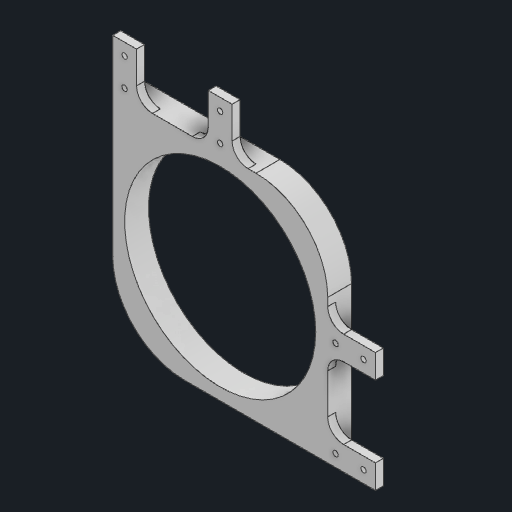
# Autodesk Inventor part: Midplate
Saved by Autodesk Inventor 2023 (Build 270158000, 158)
## iProperties
Created: 2022-11-11
Part Number: Midplate
Material: Generic
Document SubType Name: Modeling
Designer: izack
Density: 1 g/cm^3
Appearance: Default
Author: izack
Autodesk Inventor part; units mm, degrees
ref_plane "YZ Plane" through (0, 0, 0) normal (1, 0, 0) x (0, 1, 0)
ref_plane "XZ Plane" through (0, 0, 0) normal (0, 1, 0) x (-1, 0, 0)
ref_plane "XY Plane" through (0, 0, 0) normal (0, 0, 1) x (1, 0, 0)
sketch "Sketch1" plane through (0, 0, 0) normal (0, 0, 1) x (1, 0, 0)
  circle A0 centre (-0.5847, 59.562) radius 8.65 projected
  circle A1 centre (-0.5847, 59.562) radius 59.9665
  line L0 (-23.0847, -7.938) -> (21.9153, -7.938)
  line L1 (66.9153, 82.062) -> (66.9153, 82.062)
  line L2 (21.9153, 127.062) -> (21.9153, 127.062)
  line L3 (-68.0847, 82.062) -> (-68.0847, 37.062)
  line L4 (-68.0847, -7.938) -> (66.9153, 127.062) construction
  line L5 (66.9153, -7.938) -> (-68.0847, 127.062) construction
  arc A2 (-68.0847, 37.062) -> (-23.0847, -7.938) centre (-23.0847, 37.062) ccw
  arc A3 (66.9153, 82.062) -> (21.9153, 127.062) centre (21.9153, 82.062) ccw
  circle A4 centre (-0.5847, 59.562) radius 67.5
  line L6 (-18.0847, 127.062) -> (-23.0847, 127.062)
  line L7 (66.9153, 42.062) -> (66.9153, 37.062)
  arc A5 (-23.0847, 127.062) -> (-68.0847, 82.062) centre (-23.0847, 82.062) ccw
  arc A6 (21.9153, -7.938) -> (66.9153, 37.062) centre (21.9153, 37.062) ccw
  line L8 (21.9153, -7.938) -> (66.9153, -7.938)
  line L9 (66.9153, 37.062) -> (66.9153, 17.062)
  line L10 (-68.0847, 82.062) -> (-68.0847, 127.062)
  line L11 (-23.0847, 127.062) -> (-43.0847, 127.062)
  line L12 (-68.0847, 127.062) -> (-68.0847, 157.062)
  line L13 (-68.0847, 157.062) -> (-53.0847, 157.062)
  line L14 (-53.0847, 157.062) -> (-53.0847, 137.062)
  line L15 (66.9153, -7.938) -> (96.9153, -7.938)
  line L16 (96.9153, -7.938) -> (96.9153, 7.062)
  line L17 (96.9153, 7.062) -> (76.9153, 7.062)
  arc A7 (-53.0847, 137.062) -> (-43.0847, 127.062) centre (-43.0847, 137.062) ccw
  arc A8 (66.9153, 17.062) -> (76.9153, 7.062) centre (76.9153, 17.062) ccw
  line L18 (-0.5847, 59.562) -> (66.9153, 39.562) construction
  line L19 (76.9153, 67.062) -> (96.9153, 67.062)
  line L20 (96.9153, 67.062) -> (96.9153, 52.062)
  line L21 (96.9153, 52.062) -> (76.9153, 52.062)
  arc A9 (76.9153, 52.062) -> (66.9153, 42.062) centre (76.9153, 42.062) ccw
  line L22 (66.9153, 82.062) -> (66.9153, 77.062)
  arc A10 (66.9153, 77.062) -> (76.9153, 67.062) centre (76.9153, 77.062) ccw
  line L23 (-8.0847, 137.062) -> (-8.0847, 157.062)
  line L24 (-8.0847, 157.062) -> (6.9153, 157.062)
  line L25 (6.9153, 157.062) -> (6.9153, 137.062)
  arc A11 (-18.0847, 127.062) -> (-8.0847, 137.062) centre (-18.0847, 137.062) ccw
  line L26 (21.9153, 127.062) -> (16.9153, 127.062)
  arc A12 (6.9153, 137.062) -> (16.9153, 127.062) centre (16.9153, 137.062) ccw
  line L27 (-60.5847, 157.062) -> (-60.5847, 106.9366) construction
  line L28 (-0.5847, 157.062) -> (-0.5847, 127.062) construction
  line L29 (96.9153, 59.562) -> (66.9153, 59.612) construction
  line L30 (96.9153, -0.438) -> (46.9153, -0.3546) construction
  circle A13 centre (89.4153, -0.4255) radius 1.7
  circle A14 centre (71.9153, -0.3963) radius 1.7
  circle A15 centre (89.4153, 59.5745) radius 1.7
  circle A16 centre (71.9153, 59.6037) radius 1.7
  circle A17 centre (-0.5847, 132.062) radius 1.7
  circle A18 centre (-0.5847, 149.562) radius 1.7
  circle A19 centre (-60.5847, 149.562) radius 1.7
  circle A20 centre (-60.5847, 132.062) radius 1.7
  point P0 (0, 0)
  point P1 (21.9167, 127.0604)
  point P2 (66.9153, 67.062)
  point P3 (-8.0847, 127.062)
  point P4 (6.9153, 127.062)
  dimension "d0" = 119.933
  dimension "d1" = 135
  dimension "d2" = 135
  dimension "d10" = 45
  dimension "d33" = 45
  dimension "d34" = 30
  dimension "d35" = 15
  dimension "d36" = 30
  dimension "d37" = 10
  dimension "d38" = 30
  dimension "d39" = 15
  dimension "d41" = 45
  dimension "d42" = 15
  dimension "d43" = 10
  dimension "d44" = 10
  dimension "d45" = 30
  dimension "d46" = 15
  dimension "d47" = 45
  dimension "d48" = 10
  dimension "d49" = 10
  dimension "d50" = 3.4
  dimension "d51" = 3.4
  dimension "d52" = 3.4
  dimension "d53" = 3.4
  dimension "d54" = 3.4
  dimension "d55" = 3.4
  dimension "d56" = 3.4
  dimension "d57" = 3.4
  dimension "d58" = 7.5
  dimension "d59" = 25
  dimension "d60" = 7.5
  dimension "d61" = 25
  dimension "d62" = 25
  dimension "d63" = 7.5
  dimension "d64" = 7.5
  dimension "d65" = 25
  constraints: 62 end point, 30 point on line, 26 point on circle, 25 tangent, 20 centre point, 13 perpendicular, 8 midpoint, 5 horizontal, 4 parallel, 3 equal radius, 2 coincident, 2 vertical
  measures "d0" diameter of A1
  measures "d1" distance of L5.end L4.end
  measures "d2" distance of L4.end L5.start
  measures "d10" radius of A2
  measures "d33" radius of A5
  measures "d34" distance of L12.start L12.end
  measures "d35" distance of L12.end L13.end
  measures "d36" distance of L5.start L15.end
  measures "d37" radius of A7
  measures "d38" distance of point (66.915, 67.062) L19.end
  measures "d39" distance of L19.end L20.end
  measures "d41" distance between parallel lines of L21 L17
  measures "d42" distance between parallel lines of L15 L17
  measures "d43" radius of A9
  measures "d44" radius of A10
  measures "d45" distance of point (-8.085, 127.062) L23.end
  measures "d46" distance of L23.end L24.end
  measures "d47" distance between parallel lines of L14 L23
  measures "d48" radius of A11
  measures "d49" radius of A12
  measures "d50" diameter of A13
  measures "d51" diameter of A14
  measures "d52" diameter of A15
  measures "d53" diameter of A16
  measures "d54" diameter of A17
  measures "d55" diameter of A18
  measures "d56" diameter of A19
  measures "d57" diameter of A20
  measures "d58" distance from line of A13.centre L16
  measures "d59" distance from line of A14.centre L16
  measures "d60" distance from line of A15.centre L20
  measures "d61" distance from line of A16.centre L20
  measures "d62" distance from line of L24 A17.centre
  measures "d63" distance from line of L24 A18.centre
  measures "d64" distance from line of L13 A19.centre
  measures "d65" distance from line of L13 A20.centre
extrude "Extrusion1" add sketch "Sketch1" against normal blind 5 contours A2 L3 A4 L0 | A4 L3 A5 L6 A11 L23 L24 L25 A12 L26 A3 L22 A10 L19 L20 L21 A9 L7 A6 L0 | A4 | A6 L9 A8 L17 L16 L15 L8 | L10 L12 L13 L14 A7 L11 A5
sketch "Sketch2" plane through (0, 0, 0) normal (0, 0, 1) x (1, 0, 0)
  circle A0 centre (-0.5847, 59.562) radius 59.9665 projected
  circle A1 centre (-0.5847, 59.562) radius 67.5
  line L0 (96.9153, -7.938) -> (-23.0847, -7.938) projected
  line L1 (-68.0847, 127.062) -> (-68.0847, 37.062) projected
  arc A2 (-68.0847, 37.062) -> (-23.0847, -7.938) centre (-23.0847, 37.062) ccw projected
  line L2 (-23.0847, -7.938) -> (-68.0847, -7.938) projected
  circle A3 centre (-0.5847, 59.562) radius 56.9665
  line L3 (-18.0847, 127.062) -> (-43.0847, 127.062) projected
  arc A4 (-68.0847, 37.062) -> (-23.0847, -7.938) centre (-23.0847, 37.062) ccw projected
  arc A5 (66.9153, 82.062) -> (21.9153, 127.062) centre (21.9153, 82.062) ccw projected
  circle A6 centre (-0.5847, 59.562) radius 59.9665 projected
  arc A7 (76.9153, 52.062) -> (66.9153, 42.062) centre (76.9153, 42.062) ccw projected
  line L4 (76.9153, 52.062) -> (96.9153, 52.062) projected
  line L5 (96.9153, 52.062) -> (96.9153, 67.062) projected
  line L6 (96.9153, 67.062) -> (76.9153, 67.062) projected
  arc A8 (66.9153, 77.062) -> (76.9153, 67.062) centre (76.9153, 77.062) ccw projected
  line L7 (66.9153, 77.062) -> (66.9153, 82.062) projected
  line L8 (21.9153, 127.062) -> (16.9153, 127.062) projected
  arc A9 (6.9153, 137.062) -> (16.9153, 127.062) centre (16.9153, 137.062) ccw projected
  line L9 (6.9153, 137.062) -> (6.9153, 157.062) projected
  line L10 (6.9153, 157.062) -> (-8.0847, 157.062) projected
  line L11 (-8.0847, 157.062) -> (-8.0847, 137.062) projected
  arc A10 (-18.0847, 127.062) -> (-8.0847, 137.062) centre (-18.0847, 137.062) ccw projected
  line L12 (-68.0847, 157.062) -> (-68.0847, 37.062) projected
  line L13 (-23.0847, -7.938) -> (96.9153, -7.938) projected
  line L14 (96.9153, -7.938) -> (96.9153, 7.062) projected
  line L15 (96.9153, 7.062) -> (76.9153, 7.062) projected
  arc A11 (66.9153, 17.062) -> (76.9153, 7.062) centre (76.9153, 17.062) ccw projected
  line L16 (66.9153, 17.062) -> (66.9153, 42.062) projected
  arc A12 (-53.0847, 137.062) -> (-43.0847, 127.062) centre (-43.0847, 137.062) ccw projected
  line L17 (-53.0847, 137.062) -> (-53.0847, 157.062) projected
  line L18 (-53.0847, 157.062) -> (-68.0847, 157.062) projected
  arc A13 (66.9153, 17.062) -> (76.9153, 7.062) centre (76.9153, 17.062) ccw projected
  line L19 (66.9153, 17.062) -> (66.9153, -7.938)
  line L20 (76.9153, 7.062) -> (41.8417, 7.062)
  line L21 (-43.0847, 127.062) -> (-18.0847, 127.062) projected
  line L22 (16.9153, 127.062) -> (-18.0847, 127.062)
  line L23 (6.9153, 137.062) -> (6.9153, 127.062)
  arc A14 (-18.0847, 127.062) -> (-8.0847, 137.062) centre (-18.0847, 137.062) ccw projected
  line L24 (-8.0847, 137.062) -> (-8.0847, 127.062)
  arc A15 (-53.0847, 137.062) -> (-43.0847, 127.062) centre (-43.0847, 137.062) ccw projected
  line L25 (-43.0847, 127.062) -> (-68.0847, 127.062)
  line L26 (-53.0847, 137.062) -> (-53.0847, 101.9884)
  line L27 (-8.0847, 127.062) -> (-8.0847, 126.644)
  line L28 (6.9153, 127.062) -> (6.9153, 126.644)
  arc A16 (76.9153, 52.062) -> (66.9153, 42.062) centre (76.9153, 42.062) ccw projected
  line L29 (66.9153, 42.062) -> (66.9153, 77.062)
  line L30 (76.9153, 67.062) -> (66.4974, 67.062)
  line L31 (96.9153, 52.062) -> (76.9153, 52.062) projected
  line L32 (76.9153, 52.062) -> (66.4974, 52.062)
  point P0 (0, 0)
  point P1 (167.5, -7.3834)
  point P2 (-67.5, 227.6166)
  point P3 (-68.0833, 59.5604)
  point P4 (-0.5847, -7.938)
  point P5 (171.9167, -7.9396)
  point P6 (-68.0833, 222.0604)
  point P7 (21.9167, -7.9396)
  point P8 (-68.0833, 82.0604)
  point P9 (-0.5833, 127.0604)
  point P10 (-68.0847, 37.062)
  point P11 (-0.5847, -7.938)
  point P12 (-68.0847, 59.562)
  point P13 (-68.0833, 82.0604)
  point P14 (-23.0847, -7.938)
  point P15 (19.009, 124.1556)
  point P16 (-68.0847, 37.062)
  point P17 (-65.1783, 39.9683)
  point P18 (-59.0255, 46.1212)
  point P19 (12.8561, 118.0028)
  point P20 (66.9153, 59.562)
  point P21 (66.9153, -7.938)
  point P22 (-0.5847, 127.062)
  dimension "d16" = 3
  constraints: 24 end point, 7 perpendicular, 7 point on circle, 6 point on line, 6 tangent, 2 centre point, 1 coincident, 1 parallel, 4 other
  measures "d16" radial gap between concentric circles of A0 A3
extrude "Extrusion2" add sketch "Sketch2" against normal blind 10 from surface at -5 contours A1 | L29 L32 A1 | A1 L30 L29 | A1 L28 L22 L8 A5 L7 L29 L30 | L32 L29 L16 L19 L20 A1 | A1 L22 L28 | L20 L19 L0 A1 | A1 L27 L22 | L0 A2 L1 A1 | A1 L26 L25 L3 L22 L27 | L1 L25 L26 A1
body "Solid1"
